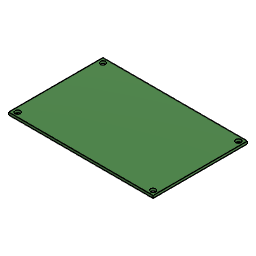
Housing Complete v6 (Autodesk Fusion 360 archive; units mm, degrees)
design "PCB Housing"
Autodesk Fusion 360 part; units mm, degrees
sketch "Sketch1" plane through (0, 0, 0) normal (0, 0, 1) x (1, 0, 0)
  line L0 (0, 0) -> (118.87, 0)
  line L1 (118.87, 0) -> (118.87, 77.597)
  line L2 (118.87, 77.597) -> (0, 77.597)
  line L3 (0, 77.597) -> (0, 0)
  circle A0 centre (3.705, 73.892) radius 3.705
  circle A1 centre (3.705, 73.892) radius 2.15
  circle A2 centre (115.165, 73.892) radius 2.15
  circle A3 centre (115.165, 73.892) radius 3.705
  circle A4 centre (115.165, 3.705) radius 3.705
  circle A5 centre (115.165, 3.705) radius 2.15
  circle A6 centre (3.705, 3.705) radius 3.705
  circle A7 centre (3.705, 3.705) radius 2.15
  dimension "d1" = 118.87
  dimension "d2" = 77.597
  dimension "d21" = 3.705
  dimension "d22" = 4.3
  constraint horizontal L0
  constraint vertical L1
  constraint horizontal L2
  constraint vertical L3
  constraint coincident L0.start L3.end
  constraint tangent L3 A0
  constraint tangent L2 A0
  constraint concentric A0 A1
  measures "d1" distance of L0.start L0.end
  measures "d2" distance of L0.start L2.end
  measures "d21" radius of A0
  measures "d22" diameter of A1
extrude "Extrude3" add sketch "Sketch1" along normal blind 2
